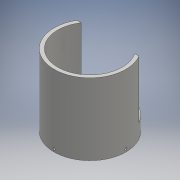
# Autodesk Inventor part: InsideCover
Saved by Autodesk Inventor 2016 (Build 200138000, 138)
## iProperties
Created: 2016-10-27
Part Number: InsideCover
Material: 一般
Document SubType Name: Modeling
Designer: Daisuke
Density: 1 g/cm^3
Appearance: 既定
Author: Daisuke
Autodesk Inventor part; units mm, degrees
ref_plane "XY Plane" through (0, 0, 0) normal (0, 0, 1) x (1, 0, 0)
sketch "スケッチ1" plane through (0, 0, 0) normal (0, 0, 1) x (1, 0, 0)
  circle A0 centre (0, 0) radius 45
  circle A1 centre (0, 0) radius 50
  dimension "d0" = 90
  dimension "d1" = 100
  constraints: 2 centre point, 2 coincident
  measures "d0" diameter of A0
  measures "d1" diameter of A1
extrude "押し出し1" add sketch "スケッチ1" along normal blind 20
sketch "スケッチ2" plane through (0, 0, 20) normal (0, 0, 1) x (1, 0, 0)
  arc A0 (-37.4166, 25) -> (37.4166, 25) centre (0, 0) ccw
  arc A1 (-43.3013, 25) -> (43.3013, 25) centre (0, 0) ccw
  line L0 (0, 0) -> (-43.3013, 25) construction
  circle A2 centre (0, 0) radius 50 construction
  line L1 (0, 0) -> (50, 0) construction
  line L2 (0, 0) -> (43.3013, 25) construction
  line L3 (0, 0) -> (50, 0) construction
  line L4 (-43.3013, 25) -> (43.3013, 25)
  dimension "d4" = 150
  dimension "d5" = 30
  constraints: 10 end point, 6 point on circle, 2 centre point, 2 coincident, 2 equal length, 2 horizontal, 2 point on line
  measures "d4" angle of L1 L0
  measures "d5" angle of L3 L2
extrude "押し出し2" add sketch "スケッチ2" along normal blind 80 contours A0 L4 A1
ref_plane "作業平面1" through (50, 0, 0) normal (1, 0, 0) x (0, 1, 0)
sketch "スケッチ3" plane through (50, 0, 0) normal (1, 0, 0) x (0, 1, 0)
  line L0 (0, 0) -> (0, 4) construction
  circle A0 centre (0, 4) radius 1.5
  dimension "d9" = 4
  dimension "d10" = 3
  constraints: 2 end point, 1 centre point, 1 coincident, 1 vertical
  measures "d9" distance of L0.start L0.end
  measures "d10" diameter of A0
extrude "押し出し3" cut sketch "スケッチ3" against normal blind 6
ref_plane "作業平面2" through (-50, 0, 0) normal (1, 0, 0) x (0, 1, 0)
ref_plane "作業平面3" through (0, 50, 0) normal (0, 1, 0) x (-1, 0, 0)
ref_plane "作業平面4" through (0, -50, 0) normal (0, 1, 0) x (-1, 0, 0)
sketch "スケッチ4" plane through (0, 50, 0) normal (0, 1, 0) x (-1, 0, 0)
  line L0 (0, 0) -> (0, 4) construction
  circle A0 centre (0, 4) radius 1.5
  dimension "d16" = 4
  dimension "d17" = 3
  constraints: 2 end point, 1 centre point, 1 coincident, 1 vertical
  measures "d16" distance of L0.start L0.end
  measures "d17" diameter of A0
extrude "押し出し4" cut sketch "スケッチ4" against normal blind 6
sketch "スケッチ5" plane through (-50, 0, 0) normal (1, 0, 0) x (0, 1, 0)
  line L0 (0, 0) -> (0, 4) construction
  circle A0 centre (0, 4) radius 1.5
  dimension "d20" = 4
  dimension "d21" = 3
  constraints: 2 end point, 1 centre point, 1 coincident, 1 vertical
  measures "d20" distance of L0.start L0.end
  measures "d21" diameter of A0
extrude "押し出し5" cut sketch "スケッチ5" along normal blind 6
sketch "スケッチ6" plane through (0, -50, 0) normal (0, 1, 0) x (-1, 0, 0)
  line L0 (0, 0) -> (0, 4) construction
  line L1 (0, 5.5) -> (0, 2.5) construction
  circle A0 centre (0, 4) radius 1.5
  dimension "d24" = 4
  dimension "d25" = 3
  constraints: 2 end point, 1 centre point, 1 coincident, 1 midpoint
  measures "d24" distance of L0.start L0.end
  measures "d25" diameter of A0
extrude "押し出し6" cut sketch "スケッチ6" along normal blind 6
